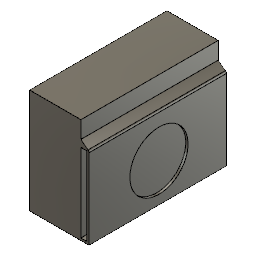
2nd mirror small calib holder v9 (Autodesk Fusion 360 design; units mm, degrees)
Autodesk Fusion 360 part; units mm, degrees
note: some values were not read from the file. Set by a fixed rule: which sketch regions a step uses.
sketch "Sketch1" plane through (0, 0, 0) normal (1, 0, 0) x (0, 0, -1)
  line L0 (0, 0) -> (-57, 0)
  line L1 (-57, 0) -> (-57, 54)
  line L2 (-57, 54) -> (0, 54)
  line L3 (0, 54) -> (0, 0)
  dimension "d1" = 57
  dimension "d2" = 54
  constraint horizontal L0
  constraint vertical L1
  constraint horizontal L2
  constraint vertical L3
  constraint coincident L0.start L3.end
  measures "d1" distance of L0.start L0.end
  measures "d2" distance of L0.start L2.end
extrude "Extrude1" add sketch "Sketch1" along normal blind 9 makes body 1
sketch "Sketch2" plane through (9, 0, 0) normal (1, 0, 0) x (0, 0, -1)
  line L0 (0, 54) -> (-57, 54)
  line L1 (-57, 54) -> (-57, 0)
  line L2 (-57, 0) -> (0, 0)
  line L3 (0, 0) -> (0, 54)
  circle A0 centre (-28, 27) radius 18.5
  circle A1 centre (-28, 27) radius 12.5
  dimension "d5" = 37
  dimension "d6" = 25
  constraint concentric A0 A1
  measures "d5" diameter of A0
  measures "d6" diameter of A1
extrude "Extrude16" cut sketch "Sketch2" against normal blind 1 contours A1 bodies 1
sketch "Sketch3" plane through (9, 27, 28) normal (1, 0, 0) x (0, 0, -1)
  line L0 (-29.01, 27.5) -> (28.01, 27.5)
  line L1 (28.01, 27.5) -> (28.01, -26.5)
  line L2 (-29.01, 27.5) -> (-29.01, -26.5)
  line L3 (28, 27) -> (-29, 27)
  line L4 (-29, 27) -> (-29, -27)
  line L5 (28, -27) -> (28, 27)
  line L6 (-30.01, 28.5) -> (-30.01, -26.5)
  line L7 (-30.01, 28.5) -> (29.01, 28.5)
  line L8 (29.01, 28.5) -> (29.01, -26.5)
  line L9 (-30.01, -26.5) -> (-29.01, -26.5)
  line L10 (29.01, -26.5) -> (28.01, -26.5)
  dimension "d7" = 0.5
  dimension "d8" = 0.01
  dimension "d9" = 0.01
  dimension "d10" = 54
  dimension "d11" = -1
  constraint horizontal L0
  constraint perpendicular L0 L1
  constraint perpendicular L0 L2
  constraint equal L1 L2
  constraint perpendicular L2 L9
  constraint perpendicular L1 L10
  measures "d7" distance of L0 L3
  measures "d8" distance of L2 L4
  measures "d9" distance of L1 L5
  measures "d10" distance of L0.start L2.end
extrude "Extrude2" add sketch "Sketch3" along normal blind -9.8 and the other way blind -0.8 separate body makes body 2
sketch "Sketch4" plane through (0, 0, -0.01) normal (0, 0, 1) x (1, 0, 0)
  line L0 (9.8, 54.5) -> (-0.8, 54.5)
  line L1 (-0.8, 54.5) -> (-0.8, 0.5)
  line L2 (-0.8, 0.5) -> (9.8, 0.5)
  line L3 (9.8, 0.5) -> (9.8, 54.5)
  line L4 (0, 54.5) -> (0, 0.5)
  line L5 (9, 0.5) -> (9, 54.5)
extrude "Extrude3" add sketch "Sketch4" along normal blind 2 contours L0 L2 L3 L5 | L0 L1 L2 L4 bodies 2
sketch "Sketch5" plane through (0, 54.5, 0) normal (0, -1, 0) x (1, 0, 0)
  line L0 (9, 1.99) -> (9.8, 1.99)
  line L1 (0, 1.99) -> (0, -0.01)
  line L2 (0, -0.01) -> (9, -0.01)
  line L3 (9.8, 1.99) -> (9.8, 57.01)
  line L4 (9.8, 57.01) -> (-0.8, 57.01)
  line L5 (-0.8, 57.01) -> (-0.8, 1.99)
  line L6 (0, 57.01) -> (0, 1.99)
  line L7 (9, -0.01) -> (9, 1.99)
  line L8 (9, 1.99) -> (9, 57.01)
  line L9 (-0.8, 1.99) -> (0, 1.99)
extrude "Extrude4" add sketch "Sketch5" along normal blind 2 contours L4 L5 L6 L9 bodies 2
sketch "Sketch6" plane through (0, 0, 57.01) normal (0, 0, -1) x (-1, 0, 0)
  line L0 (0.8, 52.5) -> (0, 52.5)
  line L1 (0, 52.5) -> (0, 54.5)
  line L2 (0, 54.5) -> (-9.8, 54.5)
  line L3 (-9.8, 54.5) -> (-9.8, 0.5)
  line L4 (-9.8, 0.5) -> (0.8, 0.5)
  line L5 (0.8, 0.5) -> (0.8, 52.5)
  line L6 (0, 0.5) -> (0, 52.5)
  line L7 (-9, 54.5) -> (-9, 0.5)
extrude "Extrude5" add sketch "Sketch6" along normal blind 2 contours L0 L4 L5 L6 | L2 L3 L4 L7 bodies 2
sketch "Sketch16" plane through (0, 55.5, 0) normal (0, 1, 0) x (-1, 0, 0)
  line L0 (-9.8, -1.01) -> (0.8, -1.01)
  line L1 (0.8, -1.01) -> (0.8, 58.01)
  line L2 (0.8, 58.01) -> (-9.8, 58.01)
  line L3 (-9.8, 58.01) -> (-9.8, -1.01)
  line L4 (-9.8, 58.01) -> (-24.8, 58.01)
  line L5 (-24.8, 58.01) -> (-24.8, -1.01)
  line L6 (-24.8, -1.01) -> (-9.8, -1.01)
  line L7 (-9.8, -1.01) -> (-9.8, 58.01)
  dimension "d81" = 15
  constraint horizontal L4
  constraint vertical L5
  constraint horizontal L6
  constraint vertical L7
  constraint coincident L2.end L3.start
  constraint coincident L0.start L3.end
  measures "d81" distance of L2.end L4.end
extrude "Extrude18" add sketch "Sketch16" against normal blind 1 contours L3 L4 L5 L6 L7 bodies 2
sketch "Sketch17" plane through (0, 54.5, 0) normal (0, -1, 0) x (1, 0, 0)
  line L0 (9.8, 55.01) -> (9, 55.01)
  line L1 (9, 55.01) -> (9, 57.01)
  line L2 (9, 57.01) -> (0, 57.01)
  line L3 (0, 57.01) -> (0, -0.01)
  line L4 (0, -0.01) -> (9, -0.01)
  line L5 (9, -0.01) -> (9, 1.99)
  line L6 (9, 1.99) -> (9.8, 1.99)
  line L7 (9.8, 1.99) -> (9.8, -1.01)
  line L8 (9.8, -1.01) -> (24.8, -1.01)
  line L9 (24.8, -1.01) -> (24.8, 58.01)
  line L10 (24.8, 58.01) -> (9.8, 58.01)
  line L11 (9.8, 58.01) -> (9.8, 55.01)
  line L12 (24.8, -1.01) -> (9.8, -1.01)
  line L13 (9.8, -1.01) -> (9.8, -0.01)
  line L14 (9.8, -0.01) -> (24.8, -0.01)
  line L15 (24.8, -0.01) -> (24.8, -1.01)
  line L16 (24.8, 58.01) -> (9.8, 58.01)
  line L17 (9.8, 58.01) -> (9.8, 57.01)
  line L18 (9.8, 57.01) -> (24.8, 57.01)
  line L19 (24.8, 57.01) -> (24.8, 58.01)
  dimension "d84" = 1
  dimension "d85" = 1
  constraint horizontal L12
  constraint vertical L13
  constraint horizontal L14
  constraint vertical L15
  constraint coincident L7 L13.end
  constraint coincident L8.end L9.start
  constraint horizontal L16
  constraint vertical L17
  constraint horizontal L18
  constraint vertical L19
  constraint coincident L11 L17.end
  constraint coincident L9.end L10.start
  measures "d84" distance of L12 L14
  measures "d85" distance of L9.end L18.end
extrude "Extrude19" add sketch "Sketch17" along normal up to surface (54 mm away) contours L9 L10 L11 L16 L17 L18 L19 | L7 L8 L9 L12 L13 L14 L15 bodies 2
sketch "Sketch19" plane through (0, 54.5, 0) normal (0, -1, 0) x (1, 0, 0)
  line L0 (24.8, -0.01) -> (23.8, -0.01)
  line L1 (23.8, -0.01) -> (23.8, 57.01)
  line L2 (23.8, 57.01) -> (24.8, 57.01)
  line L3 (24.8, 57.01) -> (24.8, -0.01)
  line L4 (21.3, 57.7) -> (19.3, 57.7)
  line L5 (19.3, 57.7) -> (19.3, -0.01)
  line L6 (19.3, -0.01) -> (21.3, -0.01)
  line L7 (21.3, -0.01) -> (21.3, 57.7)
  line L8 (24.8, 57.01) -> (9.8, 57.01)
  line L9 (9.8, 57.01) -> (9.8, 55.01)
  line L10 (9.8, 55.01) -> (9, 55.01)
  line L11 (9, 55.01) -> (9, 57.01)
  line L12 (9, 57.01) -> (0, 57.01)
  line L13 (0, 57.01) -> (0, -0.01)
  line L14 (0, -0.01) -> (9, -0.01)
  line L15 (9, -0.01) -> (9, 1.99)
  line L16 (9, 1.99) -> (9.8, 1.99)
  line L17 (9.8, 1.99) -> (9.8, -0.01)
  line L18 (9.8, -0.01) -> (24.8, -0.01)
  line L19 (24.8, -0.01) -> (24.8, 57.01)
  dimension "d89" = 1
  dimension "d90" = 2
  dimension "d91" = 2.5
  constraint horizontal L0
  constraint vertical L1
  constraint horizontal L2
  constraint vertical L3
  constraint horizontal L4
  constraint vertical L5
  constraint horizontal L6
  constraint vertical L7
  constraint collinear L2 L8
  constraint collinear L0 L18
  constraint collinear L6 L18
  constraint collinear L3 L19
  measures "d89" distance of L1 L3
  measures "d90" distance of L5 L7
  measures "d91" distance of L1 L7
extrude "Extrude20" add sketch "Sketch19" along normal blind 60 contours L0 L1 L2 L3 L8 L18 L19 | L5 L6 L7 L8 L18 bodies 2
extrude "Extrude21" cut 1 faces at (8, 28.8078, 29.8997) along direction (1, 0, 0) up to surface (1 mm away) from surface at 15.8 on bodies 1 bodies 2
sketch "Sketch25" plane through (0, 0, -0.01) normal (0, 0, 1) x (1, 0, 0)
  line L0 (21.3, 54.5) -> (21.3, 0.5)
  line L1 (21.3, 0.5) -> (23.8, 0.5)
  line L2 (23.8, 0.5) -> (23.8, 54.5)
  line L3 (23.8, 54.5) -> (21.3, 54.5)
  line L4 (24.8, 55.5) -> (24.8, 45.5)
  line L5 (24.8, 45.5) -> (21.3, 45.5)
  line L6 (21.3, 54.5) -> (21.3, 45.5)
  line L7 (24.8, 45.5) -> (24.8, 55.5)
  line L8 (24.8, 55.5) -> (24.8, 0.5)
  line L9 (-0.8, 55.5) -> (24.8, 55.5)
  line L10 (21.3, 54.5) -> (21.3, 55.5)
  line L11 (24.8, 55.5) -> (21.3, 55.5)
  line L12 (24.8, 10.5) -> (19.3, 10.5)
  line L13 (19.3, -5.5) -> (24.8, -5.5)
  line L14 (24.8, -5.5) -> (24.8, 10.5)
  line L15 (9.8, 0.5) -> (19.3, -5.5)
  line L16 (19.3, 0.5) -> (19.3, 54.5)
  line L17 (-0.8, 0.5) -> (24.8, 0.5)
  line L18 (9.8, 0.5) -> (9.8, 54.5)
  line L19 (19.3, 10.5) -> (9.8, 10.5)
  line L20 (9.8, 10.5) -> (9.8, 0.5)
  line L21 (9.8, 0.5) -> (19.3, 0.5)
  line L22 (19.3, 0.5) -> (19.3, 10.5)
  line L23 (9.8, 0.5) -> (9.8, 10.5)
  point P0 (19.3, -5.5)
  dimension "d119" = 10
  dimension "d120" = 10
  constraint coincident L0 L5.end
  constraint coincident L0.start L3.end
  constraint coincident L4.end L8
  constraint coincident L4.start L9
  constraint coincident L9 L10.end
  constraint perpendicular L9 L10
  constraint perpendicular L7 L11
  constraint horizontal L5
  constraint horizontal L12
  constraint horizontal L13
  constraint vertical L14
  constraint coincident L8 L12.start
  constraint coincident P0 L13.start
  constraint coincident L12.end L16
  constraint coincident L15.start L17
  constraint coincident L15.start L18
  constraint horizontal L19
  constraint vertical L20
  constraint horizontal L21
  constraint vertical L22
  constraint coincident L15.start L18.start
  measures "d119" distance of L5 L9
  measures "d120" distance of L12 L17
extrude "Extrude26" cut sketch "Sketch25" along normal blind 65 and the other way blind 10 contours L0 L2 L3 L5 L6 | L2 L3 L4 L5 L7 L8 L9 L10 L11 | L0 L1 L2 L12 L17 | L0 L12 L16 L17 L22 | L1 L13 L14 L15 L17 L21 | L2 L8 L12 L14 L17 | L16 L17 L18 L19 L20 L21 L22 L23 bodies 2
sketch "Sketch26" plane through (0, 0, 58.01) normal (0, 0, 1) x (1, 0, 0)
  line L0 (21.3, 55.5) -> (-0.8, 55.5)
  line L1 (-0.8, 55.5) -> (-0.8, 0.5)
  line L2 (-0.8, 0.5) -> (9.8, 0.5)
  line L3 (24.8, 10.5) -> (24.8, 45.5)
  line L4 (24.8, 45.5) -> (21.3, 45.5)
  line L5 (24.8, 45.5) -> (21.3, 45.5)
  arc A0 (21.3, 48.178) -> (24.8, 45.5) centre (41.2309, 70.6003) ccw
  line L6 (21.3, 45.5) -> (21.3, 55.5)
  line L7 (9.8, 10.5) -> (24.8, 10.5)
  line L8 (24.8, 10.5) -> (19.3, 10.5)
  line L9 (19.3, 11.5) -> (24.8, 11.5)
  line L10 (24.8, 11.5) -> (24.8, 10.5)
  line L11 (9.8, 0.5) -> (9.8, 10.5)
  line L12 (19.3, 10.5) -> (19.3, 11.5)
  dimension "d116" = 30
  dimension "d124" = 5.5
  dimension "d125" = 1
  constraint coincident L3.end L4.start
  constraint coincident L4.end L5.end
  constraint coincident L3.start L7.end
  constraint perpendicular L3 L9
  constraint perpendicular L8 L10
  constraint perpendicular L9 L12
  constraint coincident A0.start L6
  measures "d116" radius of A0
  measures "d124" distance of L10 L12
  measures "d125" distance of L8 L9
extrude "Extrude27" add sketch "Sketch26" against normal up to surface (59.02 mm away) contours L4 L5 A0 L6 | L3 L7 L8 L9 L10 L12 bodies 2
sketch "Sketch27" plane through (0, 0, 58.01) normal (0, 0, 1) x (1, 0, 0)
  arc A0 (21.3, 48.178) -> (24.8, 45.5) centre (41.2309, 70.6003) ccw
  line L0 (21.3, 48.178) -> (21.3, 55.5)
  line L1 (21.3, 55.5) -> (-0.8, 55.5)
  line L2 (-0.8, 55.5) -> (-0.8, 0.5)
  line L3 (-0.8, 0.5) -> (9.8, 0.5)
  line L4 (24.8, 10.5) -> (24.8, 45.5)
  line L5 (23.7987, 11.5) -> (21.2974, 11.5)
  line L6 (21.2974, 11.5) -> (21.2974, 45.1898)
  line L7 (21.2974, 45.1898) -> (23.7987, 45.1898)
  line L8 (23.7987, 45.1898) -> (23.7987, 11.5)
  line L9 (9.8, 0.5) -> (9.8, 10.5)
  line L10 (9.8, 10.5) -> (24.8, 10.5)
  line L11 (9.8, 10.5) -> (-0.8, 10.5)
  line L12 (-0.8, 10.5) -> (-0.8, 0.5)
  line L13 (-0.8, 0.5) -> (9.8, 0.5)
  line L14 (9.8, 0.5) -> (9.8, 10.5)
  dimension "d126" = 1
  constraint horizontal L5
  constraint vertical L6
  constraint horizontal L7
  constraint vertical L8
  constraint horizontal L11
  constraint vertical L12
  constraint horizontal L13
  constraint vertical L14
  constraint coincident L2.end L3.start
  constraint coincident L9.end L10.start
  measures "d126" distance of L5 L10
extrude "Extrude28" cut sketch "Sketch27" against normal blind 70 contours L2 L3 L9 L11 L12 L13 L14 | L5 L6 L7 L8 bodies 2
fillet "Fillet3" radius 1 1 edges at (24.8, 45.5, 28.5) on bodies 2
hidden bodies 1
equation "d9 = d8"
equation "d12 = -9 mm - edge_thickness"
equation "d14 = -edge_thickness"
equation "d16 = -edge_thickness"
equation "d17 = edge_stickout"
equation "d19 = -edge_thickness"
equation "d20 = edge_stickout"
equation "d22 = -edge_thickness"
equation "edge_thickness = 0.8 mm"
equation "edge_stickout = 2 mm"
equation "d25 = edge_stickout"
equation "d27 = -edge_thickness"
equation "d28 = -edge_thickness"
equation "d29 = -edge_thickness"
equation "slit = 2 mm"
equation "d85 = d84"
equation "d120 = d119"
